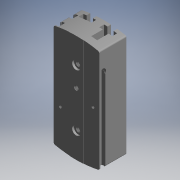
# Autodesk Inventor part: 3361863 HGPL-14-40-A-B---(GEH)
Saved by Autodesk Inventor 2017.3 (Build 213256000, 256)
## iProperties
Part Number: 3361863 HGPL-14-40-A-B---(GEH)
Material: Generic
Catalog Web Link: www.cadenas.de
Description: HGPL-B-(GEH)-Long stroke gripper
Vendor: FESTO
Document SubType Name: Modeling
Designer: partserver
Manufacturer: FESTO
Mass: 100.14 g
Surface Area: 388.313 cm^2
Volume: 100.14 cm^3
Density: 1 g/cm^3
Appearance: PSOLRGB-175-175-175
Category: PARTsolutions
Company: FESTO
Title: 3361863 HGPL-14-40-A-B
Author: Cadenas PARTsolutions
Comments: Long stroke gripper
PSOL_IDENT_0: {$CADENAS_DATA\23d-libs\festo\parts\h\hgpl\hgpl_b\parts\hgpl_b_geh.prj},198 {VTYP=3D},{NB=3361863 HG
PSOL_IDENT_1: PL-14-40-A-B---(GEH)},{LINA=3361863 HGPL-14-40-A-B},{NN=HGPL-B-(GEH)},{DATE=11.03.2020 14:57:17},{GE
PSOL_IDENT_2: OMDATE=08.01.2020 15:11:00},{VERSION=},{LINEID=10},{WBVAR=},{WBNUMERIC=}  {NB=3361863 HGPL-14-40-A-B
PSOL_IDENT_3: ---(GEH)},{LINA=3361863 HGPL-14-40-A-B},{KT=DUMMY},{TNR=3361863},{TYP=HGPL-14-40-A-B},{KDM=14},{HUB=
PSOL_IDENT_4: 40},{L21=23.600},{T8=4.500},{H10=18.000},{B1=48.000},{B100=15.000},{B2=34.500},{B20=0.250},{B3=40.00
PSOL_IDENT_5: 0},{B4=4.000},{B6=22.000},{B7=6.600},{B72=6.200},{B8=13.600},{D1=5},{D11=12.000},{D12=3.000},{D13=2.
PSOL_IDENT_6: 000},{D15=5.000},{D2=4.200},{D4=3},{D5=9.000},{D8=7.400},{E1=3.000},{EE=5.000},{H16=3.000},{H17=3.80
PSOL_IDENT_7: 0},{H18=8.800},{H2=29.000},{H3=11.200},{H6=0.000},{H7=10.000},{H8=12.000},{H9=24.400},{L1=113.600},{
PSOL_IDENT_8: L12=16.800},{L17=9.000},{L18=21.100},{L19=8.000},{L1P=67.100},{L2=0.000},{L22=0.300},{L23=18.000},{L
PSOL_IDENT_9: 2P=4.300},{L3=60.000},{L4=102},{L7=4.200},{L77=4.000},{L8=14.000},{L9=16.800},{R1=110.000},{R2=1.500
PSOL_IDENT_10: },{R7=7.500},{T1=12.500},{T3=2.100},{T5=6.500},{T7=10.000},{OBSOLETE=hier},{D10=4.200},{D14=5.200},{
PSOL_IDENT_11: D16=0.500},{L5=22},{L10=8.000},{L15=1.100},{L16=2.100},{L20=0.870},{H1=30.000},{H4=2.500},{H5=1.200}
PSOL_IDENT_12: ,{R6=0.300},{T2=1.300},{T4=5.500},{SN=4.000},{D3=5.000},{X1=0.900},{X2=1.900}
NB: 3361863 HGPL-14-40-A-B---(GEH)
NN: HGPL-B-(GEH)
NT: Long stroke gripper
NBSYN: $TNR. $TYP.---(GEH)
LINA: 3361863 HGPL-14-40-A-B
CATALOG: Festo
TNR: 3361863
TYP: HGPL-14-40-A-B
KDM: 14
L21: 23.6
T8: 4.5
B1: 48
B100: 15
B2: 34.5
B20: 0.25
B3: 40
B72: 6.2
B8: 13.6
D1: 5
D11: 12
D12: 3
D13: 2
D15: 5
D2: 4.2
D4: 3
E1: 3
EE: 5
H16: 3
H2: 29
H3: 11.2
H6: 0
H7: 10
H8: 12
H9: 24.4
L1: 113.6
L12: 16.8
L17: 9
L18: 21.1
L19: 8
L1P: 67.1
L2: 0
L22: 0.3
L23: 18
L2P: 4.3
L7: 4.2
L77: 4
L8: 14
L9: 16.8
R7: 7.5
T1: 12.5
T3: 2.1
T5: 6.5
T7: 10
OBSOLETE: hier
D10: 4.2
D14: 5.2
D16: 0.5
L5: 22
L10: 8
L15: 1.1
L16: 2.1
L20: 0.87
H4: 2.5
H5: 1.2
R6: 0.3
T2: 1.3
T4: 5.5
SN: 4
D3: 5
X1: 0.9
X2: 1.9
SUPPLIER: FESTO
ARTICLENO: 3361863 HGPL-14-40-A-B---(GEH)
BOMINFO: 3361863 HGPL-14-40-A-B
CREATOR: CADENAS GmbH
Autodesk Inventor part; units mm, degrees
sketch "Skizze_1" plane through (0, 0, 0) normal (0, 1, 0) x (-1, 0, 0)
  line L0 (24, 57.8) -> (-24, 57.8)
  line L1 (-24, 57.8) -> (-24, -57.8)
  line L2 (-24, -57.8) -> (24, -57.8)
  line L3 (24, -57.8) -> (24, 57.8)
  constraints: 8 end point
extrude "Extrusion1" add sketch "Skizze_1" along normal blind 28.8
sketch "Skizze_2" plane through (0, 0, 0) normal (0, 1, 0) x (-1, 0, 0)
  arc A0 (7.5, 56.6313) -> (-7.5, 56.6313) centre (0, -110) ccw
  line L0 (-7.5, 56.6313) -> (-7.5, -56.6313)
  arc A1 (-7.5, -56.6313) -> (7.5, -56.6313) centre (0, 110) ccw
  line L1 (7.5, -56.6313) -> (7.5, 56.6313)
  constraints: 4 end point, 4 point on circle, 2 centre point
extrude "Extrusion2" add sketch "Skizze_2" against normal blind 0.2
sketch "Sketch_25" plane through (0, -0.2, 0) normal (0, 1, 0) x (1, 0, 0)
  line L0 (-29, -61.8) -> (29, -61.8)
  line L1 (29, -61.8) -> (29, 61.8)
  line L2 (29, 61.8) -> (-29, 61.8)
  line L3 (-29, 61.8) -> (-29, -61.8)
  line L4 (-24, 52.9414) -> (-24, -52.9414)
  arc A0 (-24, -52.9414) -> (-22.8111, -54.4088) centre (-22.5, -52.9414) ccw
  arc A1 (-22.8111, -54.4088) -> (22.8111, -54.4088) centre (0, 53.2) ccw
  arc A2 (22.8111, -54.4088) -> (24, -52.9414) centre (22.5, -52.9414) ccw
  line L5 (24, -52.9414) -> (24, 52.9495)
  arc A3 (24, 52.9495) -> (22.8191, 54.4071) centre (22.51, 52.9495) ccw
  arc A4 (22.8191, 54.4071) -> (-22.8111, 54.4088) centre (0, -53.2) ccw
  arc A5 (-22.8111, 54.4088) -> (-24, 52.9414) centre (-22.5, 52.9414) ccw
  constraints: 12 end point, 12 point on circle, 6 centre point
extrude "Extrusion3" cut sketch "Sketch_25" along normal blind 29
sketch "Sketch_21" plane through (0, 0, 0) normal (1, 0, 0) x (0, 1, 0)
  line L0 (-0.2, 30) -> (28.8, 30)
  line L1 (28.8, 30) -> (28.8, 26.3)
  line L2 (28.8, 26.3) -> (18.8, 26.3)
  line L3 (18.8, 26.3) -> (18.8, 27.9)
  line L4 (18.8, 27.9) -> (14.4, 27.9)
  line L5 (14.4, 27.9) -> (14.4, 27.933)
  line L6 (14.4, 27.933) -> (2.333, 27.933)
  line L7 (2.333, 27.933) -> (1.9, 27.5)
  line L8 (1.9, 27.5) -> (1.9, 25.5)
  line L9 (1.9, 25.5) -> (-0.2, 25.5)
  line L10 (-0.2, 25.5) -> (-0.2, 30)
  line L11 (-0.2, 30) -> (28.8, 30)
  constraints: 24 end point
revolve "Revolution1" cut sketch "Sketch_21" angle 360 about axis through (0, -0.2, 30) along (0, -1, 0)
thread "Thread1" size "M5x0.8" class "6H" standard "ISO Metric profile" full length
sketch "Sketch_22" plane through (0, 0, 0) normal (1, 0, 0) x (0, 1, 0)
  line L0 (-0.2, -30) -> (28.8, -30)
  line L1 (28.8, -30) -> (28.8, -33.7)
  line L2 (28.8, -33.7) -> (18.8, -33.7)
  line L3 (18.8, -33.7) -> (18.8, -32.1)
  line L4 (18.8, -32.1) -> (14.4, -32.1)
  line L5 (14.4, -32.1) -> (14.4, -32.067)
  line L6 (14.4, -32.067) -> (2.333, -32.067)
  line L7 (2.333, -32.067) -> (1.9, -32.5)
  line L8 (1.9, -32.5) -> (1.9, -34.5)
  line L9 (1.9, -34.5) -> (-0.2, -34.5)
  line L10 (-0.2, -34.5) -> (-0.2, -30)
  line L11 (-0.2, -30) -> (28.8, -30)
  constraints: 24 end point
revolve "Revolution2" cut sketch "Sketch_22" angle 360 about axis through (0, -0.2, -30) along (0, -1, 0)
thread "Thread2" size "M5x0.8" class "6H" standard "ISO Metric profile" full length
sketch "Skizze_5" plane through (0, 0, 0) normal (0, 0, 1) x (1, 0, 0)
  line L0 (-17.8, 20) -> (-4.2, 20)
  line L1 (-4.2, 20) -> (-4.2, 25)
  line L2 (-4.2, 25) -> (-7.7, 25)
  line L3 (-7.7, 25) -> (-7.7, 33.8)
  line L4 (-7.7, 33.8) -> (7.7, 33.8)
  line L5 (7.7, 33.8) -> (7.7, 25)
  line L6 (7.7, 25) -> (4.2, 25)
  line L7 (4.2, 25) -> (4.2, 20)
  line L8 (4.2, 20) -> (17.8, 20)
  line L9 (17.8, 20) -> (17.8, 25)
  line L10 (17.8, 25) -> (14.3, 25)
  line L11 (14.3, 25) -> (14.3, 38.8)
  line L12 (14.3, 38.8) -> (-14.3, 38.8)
  line L13 (-14.3, 38.8) -> (-14.3, 25)
  line L14 (-14.3, 25) -> (-17.8, 25)
  line L15 (-17.8, 25) -> (-17.8, 20)
  constraints: 32 end point
extrude "Extrusion4" cut sketch "Skizze_5" along normal mid plane 115.6
sketch "Sketch_1" plane through (0, 0, 56.8) normal (0, 0, 1) x (1, 0, 0)
  line L0 (-26, 1.2) -> (-22.9, 1.2)
  arc A0 (-22.7, 1) -> (-22.9, 1.2) centre (-22.9, 1) ccw
  line L1 (-22.7, 1) -> (-22.7, 0.75)
  arc A1 (-22.7, 0.75) -> (-22.5, 0.55) centre (-22.5, 0.75) ccw
  line L2 (-22.5, 0.55) -> (-19.9, 0.55)
  arc A2 (-19.9, 0.55) -> (-19.5, 0.95) centre (-19.9, 0.95) ccw
  line L3 (-19.5, 0.95) -> (-19.5, 6.65)
  arc A3 (-19.5, 6.65) -> (-19.9, 7.05) centre (-19.9, 6.65) ccw
  line L4 (-19.9, 7.05) -> (-22.5, 7.05)
  arc A4 (-22.5, 7.05) -> (-22.7, 6.85) centre (-22.5, 6.85) ccw
  line L5 (-22.7, 6.85) -> (-22.7, 6.6)
  arc A5 (-22.9, 6.4) -> (-22.7, 6.6) centre (-22.9, 6.6) ccw
  line L6 (-22.9, 6.4) -> (-26, 6.4)
  line L7 (-26, 6.4) -> (-26, 1.2)
  constraints: 16 end point, 12 point on circle, 6 centre point
extrude "Extrusion5" cut sketch "Sketch_1" against normal blind 90
sketch "Sketch_2" plane through (0, 0, -33.2) normal (0, 0, 1) x (1, 0, 0)
  line L0 (-19.5, 3.8) -> (-24, 3.8)
  line L1 (-24, 3.8) -> (-24, 7.3)
  line L2 (-24, 7.3) -> (-19.5, 7.3)
  line L3 (-19.5, 7.3) -> (-19.5, 3.8)
  line L4 (-19.5, 3.8) -> (-24, 3.8)
  constraints: 10 end point
revolve "Revolution3" cut sketch "Sketch_2" angle 360 about axis through (-19.5, 3.8, -33.2) along (1, 0, 0)
sketch "Skizze_7" plane through (0, 24.2, 0) normal (0, 1, 0) x (1, 0, 0)
  line L0 (-20, -54.9665) -> (-20, -45.8067)
  line L1 (-20, -45.8067) -> (-18.7705, -46.5165)
  line L2 (-18.7705, -46.5165) -> (-18.7705, -54.696)
  line L3 (-18.7705, -54.696) -> (-18.5, -54.9665)
  line L4 (-18.5, -54.9665) -> (-18.5, -55.9665)
  line L5 (-18.5, -55.9665) -> (-20, -55.9665)
  line L6 (-20, -55.9665) -> (-20, -45.8067)
  constraints: 14 end point
revolve "Revolution4" cut sketch "Skizze_7" angle 360 about axis through (-20, 24.2, 54.9665) along (0, 0, 1)
thread "Thread3" size "M3x0.5" class "6H" standard "ISO Metric profile" length 6.2295
sketch "Skizze_8" plane through (0, 24.2, 0) normal (0, 1, 0) x (1, 0, 0)
  line L0 (20, -54.9665) -> (20, -45.8067)
  line L1 (20, -45.8067) -> (21.2295, -46.5165)
  line L2 (21.2295, -46.5165) -> (21.2295, -54.696)
  line L3 (21.2295, -54.696) -> (21.5, -54.9665)
  line L4 (21.5, -54.9665) -> (21.5, -55.9665)
  line L5 (21.5, -55.9665) -> (20, -55.9665)
  line L6 (20, -55.9665) -> (20, -45.8067)
  constraints: 14 end point
revolve "Revolution5" cut sketch "Skizze_8" angle 360 about axis through (20, 24.2, 54.9665) along (0, 0, 1)
thread "Thread4" size "M3x0.5" class "6H" standard "ISO Metric profile" length 6.2295
sketch "Skizze_9" plane through (0, 0, 0) normal (1, 0, 0) x (0, 1, 0)
  line L0 (9.8, 47.4235) -> (9.8, 56.8)
  line L1 (9.8, 56.8) -> (11.3, 56.8)
  line L2 (11.3, 56.8) -> (11.0295, 56.5295)
  line L3 (11.0295, 56.5295) -> (11.0295, 48.1333)
  line L4 (11.0295, 48.1333) -> (9.8, 47.4235)
  line L5 (9.8, 47.4235) -> (9.8, 56.8)
  constraints: 12 end point
revolve "Revolution6" cut sketch "Skizze_9" angle 360 about axis through (0, 9.8, 47.4235) along (0, 0, -1)
thread "Thread5" size "M3x0.5" class "6H" standard "ISO Metric profile" length 6.2295
sketch "Skizze_10" plane through (0, 0, 0) normal (1, 0, 0) x (0, 1, 0)
  line L0 (21.8, 47.4235) -> (21.8, 56.8)
  line L1 (21.8, 56.8) -> (23.3, 56.8)
  line L2 (23.3, 56.8) -> (23.0295, 56.5295)
  line L3 (23.0295, 56.5295) -> (23.0295, 48.1333)
  line L4 (23.0295, 48.1333) -> (21.8, 47.4235)
  line L5 (21.8, 47.4235) -> (21.8, 56.8)
  constraints: 12 end point
revolve "Revolution7" cut sketch "Skizze_10" angle 360 about axis through (0, 21.8, 47.4235) along (0, 0, -1)
thread "Thread6" size "M3x0.5" class "6H" standard "ISO Metric profile" length 6.2295
sketch "Sketch13" plane through (24, 0, -52.9495) normal (1, 0, 0) x (0, 0, -1)
  point P0 (-52.9495, 11)
hole "Hole1" at (24, 11, 0) direction (-1, 0, 0) diameter 4.134 depth 5.2 tip angle 120 countersink diameter 5 countersink angle 90 thread size "M5x0.8" class "6H" standard "ISO Metric profile"
sketch "Sketch14" plane through (24, 0, -52.9495) normal (1, 0, 0) x (0, 0, -1)
  point P0 (-69.7495, 11)
hole "Hole2" at (24, 11, 16.8) direction (-1, 0, 0) diameter 4.134 depth 5.2 tip angle 120 countersink diameter 5 countersink angle 90 thread size "M5x0.8" class "6H" standard "ISO Metric profile"
sketch "Skizze_15" plane through (0, 0, 0) normal (0, 0, 1) x (1, 0, 0)
  line L0 (-17.5, 0) -> (-17.5, 3)
  line L1 (-17.5, 3) -> (-16.2705, 3)
  line L2 (-16.2705, 3) -> (-16.2705, 0.2705)
  line L3 (-16.2705, 0.2705) -> (-16, 0)
  line L4 (-16, 0) -> (-17.5, 0)
  line L5 (-17.5, 0) -> (-17.5, 3)
  constraints: 12 end point
revolve "Revolution8" cut sketch "Skizze_15" angle 360 about axis through (-17.5, 0, 0) along (0, -1, 0)
thread "Thread7" size "M3x0.5" class "6H" standard "ISO Metric profile" full length
sketch "Skizze_16" plane through (0, 0, 16.8) normal (0, 0, 1) x (1, 0, 0)
  line L0 (17, 0) -> (17, 3)
  line L1 (17, 3) -> (18.2295, 3)
  line L2 (18.2295, 3) -> (18.2295, 0.2705)
  line L3 (18.2295, 0.2705) -> (18.5, 0)
  line L4 (18.5, 0) -> (17, 0)
  line L5 (17, 0) -> (17, 3)
  constraints: 12 end point
revolve "Revolution9" cut sketch "Skizze_16" angle 360 about axis through (17, 0, 16.8) along (0, -1, 0)
thread "Thread8" size "M3x0.5" class "6H" standard "ISO Metric profile" full length
sketch "Sketch_4" plane through (0, 0, 0) normal (1, 0, 0) x (0, 1, 0)
  line L0 (28.6, 0) -> (29, 0)
  line L1 (29, 0) -> (29, -6)
  line L2 (29, -6) -> (28.3, -6)
  line L3 (28.3, -6) -> (28.6, -5.7)
  line L4 (28.6, -5.7) -> (28.6, 0)
  line L5 (28.6, 0) -> (29, 0)
  constraints: 12 end point
revolve "Revolution10" cut sketch "Sketch_4" angle 360 about axis through (0, 28.6, 0) along (0, -1, 0)
sketch "Sketch_6" plane through (0, 0, 0) normal (1, 0, 0) x (0, 1, 0)
  line L0 (-0.2, -9) -> (28.8, -9)
  line L1 (28.8, -9) -> (28.8, -11.5)
  line L2 (28.8, -11.5) -> (28.367, -11.067)
  line L3 (28.367, -11.067) -> (0.233, -11.067)
  line L4 (0.233, -11.067) -> (-0.2, -11.5)
  line L5 (-0.2, -11.5) -> (-0.2, -9)
  line L6 (-0.2, -9) -> (28.8, -9)
  constraints: 14 end point
revolve "Revolution11" cut sketch "Sketch_6" angle 360 about axis through (0, -0.2, -9) along (0, -1, 0)
thread "Thread9" size "M5x0.8" class "6H" standard "ISO Metric profile" length 5.517
thread "Thread10" size "M5x0.8" class "6H" standard "ISO Metric profile" length 5.567
sketch "Sketch_7" plane through (0, 0, 0) normal (1, 0, 0) x (0, 1, 0)
  line L0 (26.7226, -4) -> (28.8, -4)
  line L1 (28.8, -4) -> (28.8, -5)
  line L2 (28.8, -5) -> (27.3, -5)
  line L3 (27.3, -5) -> (26.7226, -4)
  line L4 (26.7226, -4) -> (28.8, -4)
  constraints: 10 end point
revolve "Revolution12" cut sketch "Sketch_7" angle 360 about axis through (0, 26.7226, -4) along (0, -1, 0)
sketch "Sketch_8" plane through (0, 0, 0) normal (1, 0, 0) x (0, 1, 0)
  line L0 (26.7226, 4) -> (28.8, 4)
  line L1 (28.8, 4) -> (28.8, 3)
  line L2 (28.8, 3) -> (27.3, 3)
  line L3 (27.3, 3) -> (26.7226, 4)
  line L4 (26.7226, 4) -> (28.8, 4)
  constraints: 10 end point
revolve "Revolution13" cut sketch "Sketch_8" angle 360 about axis through (0, 26.7226, 4) along (0, -1, 0)
sketch "Sketch_9" plane through (0, 0, 0) normal (1, 0, 0) x (0, 1, 0)
  line L0 (25, 0) -> (28.6, 0)
  line L1 (28.6, 0) -> (28.6, -1.5)
  line L2 (28.6, -1.5) -> (25, -1.5)
  line L3 (25, -1.5) -> (25, 0)
  line L4 (25, 0) -> (28.6, 0)
  constraints: 10 end point
revolve "Revolution14" cut sketch "Sketch_9" angle 360 about axis through (0, 25, 0) along (0, -1, 0)
sketch "Sketch_10" plane through (0, 0, 11.8) normal (0, 0, 1) x (1, 0, 0)
  line L0 (4.2, 25) -> (4.2, 20)
  line L1 (4.2, 20) -> (7.9, 20)
  line L2 (7.9, 20) -> (7.9, 7.7)
  line L3 (7.9, 7.7) -> (14.1, 7.7)
  line L4 (14.1, 7.7) -> (14.1, 20)
  line L5 (14.1, 20) -> (17.8, 20)
  line L6 (17.8, 20) -> (17.8, 25)
  line L7 (17.8, 25) -> (14.3, 25)
  line L8 (14.3, 25) -> (14.3, 28.8)
  line L9 (14.3, 28.8) -> (7.7, 28.8)
  line L10 (7.7, 28.8) -> (7.7, 25)
  line L11 (7.7, 25) -> (4.2, 25)
  constraints: 24 end point
extrude "Extrusion6" cut sketch "Sketch_10" along normal blind 113.6
sketch "Sketch_11" plane through (0, 0, -11.8) normal (0, 0, 1) x (1, 0, 0)
  line L0 (-17.8, 25) -> (-17.8, 20)
  line L1 (-17.8, 20) -> (-14.1, 20)
  line L2 (-14.1, 20) -> (-14.1, 7.7)
  line L3 (-14.1, 7.7) -> (-7.9, 7.7)
  line L4 (-7.9, 7.7) -> (-7.9, 20)
  line L5 (-7.9, 20) -> (-4.2, 20)
  line L6 (-4.2, 20) -> (-4.2, 25)
  line L7 (-4.2, 25) -> (-7.7, 25)
  line L8 (-7.7, 25) -> (-7.7, 28.8)
  line L9 (-7.7, 28.8) -> (-14.3, 28.8)
  line L10 (-14.3, 28.8) -> (-14.3, 25)
  line L11 (-14.3, 25) -> (-17.8, 25)
  constraints: 24 end point
extrude "Extrusion7" cut sketch "Sketch_11" against normal blind 113.6
sketch "Sketch_12" plane through (11, 0, 0) normal (1, 0, 0) x (0, 0, -1)
  line L0 (45, 10.8) -> (-11.8, 10.8)
  line L1 (-11.8, 10.8) -> (-11.8, 13.3)
  line L2 (-11.8, 13.3) -> (-2.5733, 13.3)
  line L3 (-2.5733, 13.3) -> (-2.5733, 18.3)
  line L4 (-2.5733, 18.3) -> (45, 18.3)
  line L5 (45, 18.3) -> (45, 10.8)
  line L6 (45, 10.8) -> (-11.8, 10.8)
  constraints: 14 end point
revolve "Revolution15" cut sketch "Sketch_12" angle 360 about axis through (11, 10.8, -45) along (0, 0, -1)
sketch "Sketch_14" plane through (-11, 0, 0) normal (1, 0, 0) x (0, 0, -1)
  line L0 (11.8, 10.8) -> (-45, 10.8)
  line L1 (-45, 10.8) -> (-45, 18.3)
  line L2 (-45, 18.3) -> (2.5733, 18.3)
  line L3 (2.5733, 18.3) -> (2.5733, 13.3)
  line L4 (2.5733, 13.3) -> (11.8, 13.3)
  line L5 (11.8, 13.3) -> (11.8, 10.8)
  line L6 (11.8, 10.8) -> (-45, 10.8)
  constraints: 14 end point
revolve "Revolution16" cut sketch "Sketch_14" angle 360 about axis through (-11, 10.8, -11.8) along (0, 0, -1)
sketch "Sketch_15" plane through (0, 0, -56.8) normal (0, 0, 1) x (1, 0, 0)
  line L0 (19.5, 21.05) -> (19.5, 15.35)
  arc A0 (19.5, 15.35) -> (19.9, 14.95) centre (19.9, 15.35) ccw
  line L1 (19.9, 14.95) -> (22.5, 14.95)
  arc A1 (22.5, 14.95) -> (22.7, 15.15) centre (22.5, 15.15) ccw
  line L2 (22.7, 15.15) -> (22.7, 15.4)
  arc A2 (22.9, 15.6) -> (22.7, 15.4) centre (22.9, 15.4) ccw
  line L3 (22.9, 15.6) -> (26, 15.6)
  line L4 (26, 15.6) -> (26, 6.8)
  line L5 (26, 6.8) -> (22.9, 6.8)
  arc A3 (22.7, 7) -> (22.9, 6.8) centre (22.9, 7) ccw
  line L6 (22.7, 7) -> (22.7, 7.25)
  arc A4 (22.7, 7.25) -> (22.5, 7.45) centre (22.5, 7.25) ccw
  line L7 (22.5, 7.45) -> (19.9, 7.45)
  arc A5 (19.9, 7.45) -> (19.5, 7.05) centre (19.9, 7.05) ccw
  line L8 (19.5, 7.05) -> (19.5, 1.35)
  arc A6 (19.5, 1.35) -> (19.9, 0.95) centre (19.9, 1.35) ccw
  line L9 (19.9, 0.95) -> (22.5, 0.95)
  arc A7 (22.5, 0.95) -> (22.7, 1.15) centre (22.5, 1.15) ccw
  line L10 (22.7, 1.15) -> (22.7, 1.4)
  arc A8 (22.9, 1.6) -> (22.7, 1.4) centre (22.9, 1.4) ccw
  line L11 (22.9, 1.6) -> (31, 1.6)
  line L12 (31, 1.6) -> (31, 20.8)
  line L13 (31, 20.8) -> (22.9, 20.8)
  arc A9 (22.7, 21) -> (22.9, 20.8) centre (22.9, 21) ccw
  line L14 (22.7, 21) -> (22.7, 21.25)
  arc A10 (22.7, 21.25) -> (22.5, 21.45) centre (22.5, 21.25) ccw
  line L15 (22.5, 21.45) -> (19.9, 21.45)
  arc A11 (19.9, 21.45) -> (19.5, 21.05) centre (19.9, 21.05) ccw
  constraints: 32 end point, 24 point on circle, 12 centre point
extrude "Extrusion8" cut sketch "Sketch_15" along normal blind 90
sketch "Sketch_16" plane through (0, 0, 33.2) normal (0, 0, 1) x (1, 0, 0)
  line L0 (24, 4) -> (19.5, 4)
  line L1 (19.5, 4) -> (19.5, 7.5)
  line L2 (19.5, 7.5) -> (24, 7.5)
  line L3 (24, 7.5) -> (24, 4)
  line L4 (24, 4) -> (19.5, 4)
  constraints: 10 end point
revolve "Revolution17" cut sketch "Sketch_16" angle 360 about axis through (24, 4, 33.2) along (1, 0, 0)
sketch "Sketch_17" plane through (0, 0, 33.2) normal (0, 0, 1) x (1, 0, 0)
  line L0 (24, 18) -> (19.5, 18)
  line L1 (19.5, 18) -> (19.5, 21.5)
  line L2 (19.5, 21.5) -> (24, 21.5)
  line L3 (24, 21.5) -> (24, 18)
  line L4 (24, 18) -> (19.5, 18)
  constraints: 10 end point
revolve "Revolution18" cut sketch "Sketch_17" angle 360 about axis through (24, 18, 33.2) along (1, 0, 0)
ref_plane "GEH_XY" through (0, 0, 0) normal (0, 1, 0) x (1, 0, 0)
ref_plane "GEH_YZ" through (0, 0, 0) normal (1, 0, 0) x (0, 0, -1)
ref_plane "GEH_ZX" through (0, 0, 0) normal (0, 0, -1) x (0, 1, 0)
ref_plane "HUBRED_XY" through (0, 10, 57.8) normal (0, 0, 1) x (1, 0, 0)
ref_plane "HUBRED_YZ" through (0, 10, 57.8) normal (1, 0, 0) x (0, 1, 0)
ref_plane "HUBRED_ZX" through (0, 10, 57.8) normal (0, 1, 0) x (0, 0, 1)
ref_plane "JAW1_XY" through (-11, 10.8, 45) normal (0, 0, 1) x (1, 0, 0)
ref_plane "JAW1_YZ" through (-11, 10.8, 45) normal (1, 0, 0) x (0, 1, 0)
ref_plane "JAW1_ZX" through (-11, 10.8, 45) normal (0, 1, 0) x (0, 0, 1)
ref_plane "JAW2_XY" through (11, 10.8, -45) normal (0, 0, 1) x (1, 0, 0)
ref_plane "JAW2_YZ" through (11, 10.8, -45) normal (1, 0, 0) x (0, 1, 0)
ref_plane "JAW2_ZX" through (11, 10.8, -45) normal (0, 1, 0) x (0, 0, 1)
ref_plane "NIPPEL_XY" through (0, -9.8667, -9) normal (0, 1, 0) x (1, 0, 0)
ref_plane "NIPPEL_YZ" through (0, -9.8667, -9) normal (1, 0, 0) x (0, 0, -1)
ref_plane "NIPPEL_ZX" through (0, -9.8667, -9) normal (0, 0, -1) x (0, 1, 0)
ref_plane "NIPPEL_OBEN_XY" through (0, 29.2, -9) normal (0, -1, 0) x (1, 0, 0)
ref_plane "NIPPEL_OBEN_YZ" through (0, 29.2, -9) normal (1, 0, 0) x (0, 0, 1)
ref_plane "NIPPEL_OBEN_ZX" through (0, 29.2, -9) normal (0, 0, 1) x (0, -1, 0)
ref_plane "NIPPEL_UNTEN_XY" through (0, -0.2, -9) normal (0, 1, 0) x (1, 0, 0)
ref_plane "NIPPEL_UNTEN_YZ" through (0, -0.2, -9) normal (1, 0, 0) x (0, 0, -1)
ref_plane "NIPPEL_UNTEN_ZX" through (0, -0.2, -9) normal (0, 0, -1) x (0, 1, 0)
ref_plane "PIN_1_XY" through (17, 0, 16.8) normal (0, -1, 0) x (1, 0, 0)
ref_plane "PIN_1_YZ" through (17, 0, 16.8) normal (1, 0, 0) x (0, 0, 1)
ref_plane "PIN_1_ZX" through (17, 0, 16.8) normal (0, 0, 1) x (0, -1, 0)
ref_plane "PIN_2_XY" through (-17.5, 0, 0) normal (0, -1, 0) x (1, 0, 0)
ref_plane "PIN_2_YZ" through (-17.5, 0, 0) normal (1, 0, 0) x (0, 0, 1)
ref_plane "PIN_2_ZX" through (-17.5, 0, 0) normal (0, 0, 1) x (0, -1, 0)
ref_plane "ZBH_UNTEN_1_XY" through (0, 1.9, -30) normal (0, 1, 0) x (1, 0, 0)
ref_plane "ZBH_UNTEN_1_YZ" through (0, 1.9, -30) normal (1, 0, 0) x (0, 0, -1)
ref_plane "ZBH_UNTEN_1_ZX" through (0, 1.9, -30) normal (0, 0, -1) x (0, 1, 0)
ref_plane "ZBH_UNTEN_2_XY" through (0, 1.9, 30) normal (0, 1, 0) x (1, 0, 0)
ref_plane "ZBH_UNTEN_2_YZ" through (0, 1.9, 30) normal (1, 0, 0) x (0, 0, -1)
ref_plane "ZBH_UNTEN_2_ZX" through (0, 1.9, 30) normal (0, 0, -1) x (0, 1, 0)
body "Solid1"
